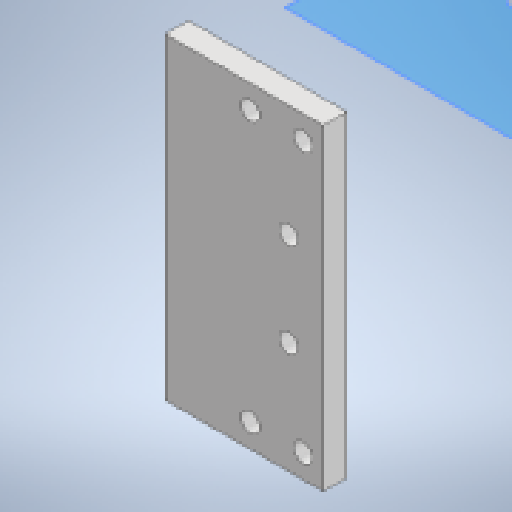
# Autodesk Inventor part: кыша_каретки
Saved by Autodesk Inventor 2023.1 (Build 271208000, 208)
## iProperties
Created: 2026-01-16
Part Number: кыша_каретки
Material: Типовые
Document SubType Name: Modeling
Designer: DELL
Density: 1 g/cm^3
Appearance: По умолчанию
Author: DELL
Autodesk Inventor part; units mm, degrees
ref_plane "YZ Plane" through (0, 0, 0) normal (1, 0, 0) x (0, 1, 0)
ref_plane "XZ Plane" through (0, 0, 0) normal (0, 1, 0) x (-1, 0, 0)
ref_plane "XY Plane" through (0, 0, 0) normal (0, 0, 1) x (1, 0, 0)
sketch "Эскиз1" plane through (0, 0, 0) normal (0, 0, 1) x (1, 0, 0)
  line L0 (-8, 5) -> (8, 5) construction
  line L1 (8, 5) -> (8, -3) construction
  circle A0 centre (2, -30) radius 1.75 construction
  circle A1 centre (2, -14) radius 1.75 construction
  line L2 (-19, 5) -> (-19, -62) construction
  line L3 (8, 5) -> (-19, 5)
  line L4 (-19, 5) -> (-19, -49)
  line L5 (-19, -49) -> (8, -49)
  line L6 (8, -49) -> (8, 5)
  circle A2 centre (2, -30) radius 1.6
  circle A3 centre (2, -14) radius 1.6
  circle A4 centre (-4.5, -45) radius 2.1 construction
  circle A5 centre (4.5, -45) radius 2.1 construction
  circle A6 centre (-4.5, 1) radius 2.1 construction
  circle A7 centre (4.5, 1) radius 2.1 construction
  circle A8 centre (-4.5, 1) radius 1.6
  circle A9 centre (4.5, 1) radius 1.6
  circle A10 centre (-4.5, -45) radius 1.6
  circle A11 centre (4.5, -45) radius 1.6
  point P0 (0, 0)
  dimension "d0" = 3.2
  dimension "d1" = 3.2
  dimension "d2" = 19
  dimension "d3" = 3.2
  dimension "d4" = 3.2
  dimension "d5" = 3.2
  dimension "d6" = 3.2
  constraints: 8 end point, 6 centre point, 6 coincident, 2 parallel, 1 horizontal, 1 perpendicular, 1 point on line
  measures "d0" diameter of A2
  measures "d1" diameter of A3
  measures "d2" distance from line of L5 A2.centre
  measures "d3" diameter of A8
  measures "d4" diameter of A9
  measures "d5" diameter of A10
  measures "d6" diameter of A11
extrude "Выдавливание1" add sketch "Эскиз1" along normal blind 4
